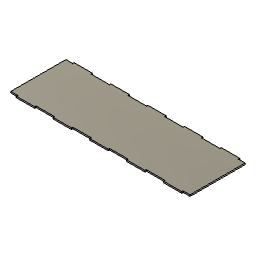
Banda version 2 v3 (Autodesk Fusion 360 archive; units mm, degrees)
design "Parte Superior"
Autodesk Fusion 360 part; units mm, degrees
sketch "Boceto1" plane through (0, 0, 0) normal (0, 0, 1) x (1, 0, 0)
  line L0 (-195, 0) -> (-195, -60)
  line L1 (-100, -60) -> (-100, -63)
  line L2 (-100, -63) -> (-60, -63)
  line L3 (-60, -63) -> (-60, -60)
  line L4 (-60, -60) -> (-20, -60)
  line L5 (-20, -60) -> (-20, -63)
  line L6 (-20, -63) -> (0, -63)
  line L7 (0, 0) -> (-195, 0) construction
  line L8 (-100, 60) -> (-100, 63)
  line L9 (-100, 63) -> (-60, 63)
  line L10 (-20, 60) -> (-20, 63)
  line L11 (-60, 60) -> (-20, 60)
  line L12 (-60, 63) -> (-60, 60)
  line L13 (-20, 63) -> (0, 63)
  line L14 (-195, 0) -> (-195, 60)
  line L15 (0, -63) -> (0, 63) construction
  line L16 (0, -63) -> (0, 63) construction
  line L17 (-100, -60) -> (-140, -60)
  line L18 (-140, -60) -> (-140, -63)
  line L19 (-140, -63) -> (-180, -63)
  line L20 (-180, -63) -> (-180, -60)
  line L21 (-180, -60) -> (-195, -60)
  line L22 (-100, 60) -> (-140, 60)
  line L23 (-140, 60) -> (-140, 63)
  line L24 (-140, 63) -> (-180, 63)
  line L25 (-180, 63) -> (-180, 60)
  line L26 (-180, 60) -> (-195, 60)
  line L27 (60, -60) -> (20, -60)
  line L28 (100, 63) -> (60, 63)
  line L29 (60, 60) -> (20, 60)
  line L30 (0, 0) -> (195, 0) construction
  line L31 (20, 60) -> (20, 63)
  line L32 (20, 63) -> (0, 63)
  line L33 (140, -63) -> (180, -63)
  line L34 (180, -63) -> (180, -60)
  line L35 (180, -60) -> (195, -60)
  line L36 (195, 0) -> (195, -60)
  line L37 (195, 0) -> (195, 60)
  line L38 (180, 60) -> (195, 60)
  line L39 (180, 63) -> (180, 60)
  line L40 (140, 63) -> (180, 63)
  line L41 (100, -60) -> (140, -60)
  line L42 (100, -63) -> (60, -63)
  line L43 (20, -63) -> (0, -63)
  line L44 (100, 60) -> (140, 60)
  line L45 (140, 60) -> (140, 63)
  line L46 (100, -60) -> (100, -63)
  line L47 (140, -60) -> (140, -63)
  line L48 (20, -63) -> (20, -60)
  line L49 (60, -63) -> (60, -60)
  line L50 (100, 63) -> (100, 60)
  line L51 (60, 63) -> (60, 60)
  point P0 (0, 63)
  dimension "d2" = 195
  dimension "d4" = 20
  dimension "d6" = 40
  dimension "d7" = 3
  dimension "d8" = 3
  dimension "d9" = 3
  dimension "d10" = 60
  dimension "d13" = 40
  dimension "d14" = 40
  dimension "d15" = 3
  dimension "d16" = 40
  dimension "d17" = 3
  dimension "d18" = 40
  dimension "d19" = 3
  dimension "d20" = 40
  dimension "d21" = 3
  constraint vertical L0
  constraint perpendicular L1 L2
  constraint perpendicular L2 L3
  constraint perpendicular L3 L4
  constraint perpendicular L4 L5
  constraint perpendicular L5 L6
  constraint coincident L7.start L30.start
  constraint perpendicular L0 L7
  constraint symmetric L0.start L7 L14.start
  constraint symmetric L0.end L7 L14.end
  constraint symmetric L1.start L7 L8.start
  constraint symmetric L1.end L7 L8.end
  constraint symmetric L2.end L7 L9.end
  constraint symmetric L3.end L7 L11.start
  constraint symmetric L4.end L7 L10.start
  constraint symmetric L5.end L7 L10.end
  constraint symmetric P0 L15 L13.end
  constraint perpendicular L1 L17
  constraint perpendicular L17 L18
  constraint perpendicular L18 L19
  constraint perpendicular L19 L20
  constraint perpendicular L0 L21
  constraint perpendicular L8 L22
  constraint perpendicular L22 L23
  constraint perpendicular L23 L24
  constraint perpendicular L24 L25
  constraint symmetric L0.start L15 L30.end
  constraint symmetric L0.end L15 L35.end
  constraint symmetric L1.start L15 L41.start
  constraint symmetric L1.end L15 L42.start
  constraint symmetric L2.end L15 L42.end
  constraint symmetric L3.end L15 L27.start
  constraint symmetric L4.end L15 L27.end
  constraint symmetric L5.end L15 L43.start
  constraint symmetric L6.end L15 L16.start
  constraint symmetric L7.start L15 L30.start
  constraint symmetric L8.start L15 L44.start
  constraint symmetric L11.start L15 L29.start
  constraint symmetric L9.end L15 L28.end
  constraint symmetric L8.end L15 L28.start
  constraint symmetric L10.start L15 L29.end
  constraint symmetric L14.end L15 L37.end
  constraint symmetric L10.end L15 L31.end
  constraint symmetric L15 P0 L13.end
  constraint symmetric L15 L17.end L41.end
  constraint symmetric L15 L18.end L33.start
  constraint symmetric L15 L19.end L33.end
  constraint symmetric L15 L20.end L34.end
  constraint symmetric L15 L22.end L44.end
  constraint symmetric L15 L23.end L40.start
  constraint symmetric L15 L24.end L39.start
  constraint symmetric L15 L25.end L38.start
  measures "d2" distance of L0.start L7.start
  measures "d4" distance of L5.end L6.end
  measures "d6" distance of L1.end L2.end
  measures "d7" distance of L1.start L1.end
  measures "d8" distance of L2.end L3.end
  measures "d9" distance of L4.end L5.end
  measures "d10" distance of L0.start L0.end
  measures "d13" distance of L3.end L4.end
  measures "d14" distance of L1.start L17.end
  measures "d15" distance of L17.end L18.end
  measures "d16" distance of L18.end L19.end
  measures "d17" distance of L19.end L20.end
  measures "d18" distance of L8.start L22.end
  measures "d19" distance of L22.end L23.end
  measures "d20" distance of L23.end L24.end
  measures "d21" distance of L24.end L25.end
extrude "Extruir2" add sketch "Boceto1" along normal blind 3

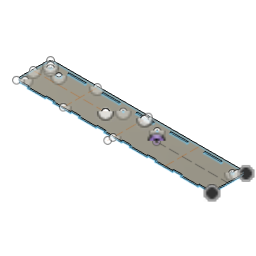
design "Lateral son motor"
Autodesk Fusion 360 part; units mm, degrees
sketch "Boceto1" plane through (0, 0, 0) normal (0, 0, 1) x (1, 0, 0)
  line L0 (-60.0005, 40.4137) -> (-60.0005, -55) construction
  line L1 (169.9995, -29.5863) -> (169.9995, 30.4137)
  line L2 (159.9995, 40.4137) -> (-60.0005, 40.4137)
  line L3 (0, 0) -> (169.9995, 0) construction
  line L4 (-0.0005, 34.4137) -> (39.9995, 34.4137)
  line L5 (39.9995, 34.4137) -> (39.9995, 31.4137)
  line L6 (39.9995, 31.4137) -> (-0.0005, 31.4137)
  line L7 (-0.0005, 31.4137) -> (-0.0005, 34.4137)
  line L8 (-60.0005, 34.4137) -> (-40.0005, 34.4137)
  line L9 (-40.0005, 34.4137) -> (-40.0005, 31.4137)
  line L10 (-40.0005, 31.4137) -> (-60.0005, 31.4137)
  circle A0 centre (-20.0005, 21.4137) radius 1
  circle A1 centre (153.9995, 24.4137) radius 2.5
  arc A2 (169.9995, 30.4137) -> (159.9995, 40.4137) centre (159.9995, 30.4137) ccw
  line L11 (79.9995, -39.5863) -> (79.9995, -42.5863)
  line L12 (79.9995, -42.5863) -> (39.9995, -42.5863)
  line L13 (39.9995, -42.5863) -> (39.9995, -39.5863)
  line L14 (39.9995, -39.5863) -> (19.9995, -39.5863)
  line L15 (19.9995, -39.5863) -> (19.9995, -42.5863)
  line L16 (19.9995, -42.5863) -> (-20.0005, -42.5863)
  line L17 (-20.0005, -42.5863) -> (-20.0005, -39.5863)
  line L18 (-20.0005, -39.5863) -> (-40.0005, -39.5863)
  line L19 (-40.0005, -39.5863) -> (-40.0005, -42.5863)
  line L20 (-40.0005, -42.5863) -> (-60.0005, -42.5863)
  line L21 (79.9995, -39.5863) -> (99.9995, -39.5863)
  line L22 (99.9995, -39.5863) -> (99.9995, -42.5863)
  line L23 (99.9995, -42.5863) -> (139.9995, -42.5863)
  line L24 (139.9995, -42.5863) -> (139.9995, -39.5863)
  line L25 (139.9995, -39.5863) -> (159.9995, -39.5863)
  arc A3 (159.9995, -39.5863) -> (169.9995, -29.5863) centre (159.9995, -29.5863) ccw
  line L26 (59.9995, 40.4137) -> (59.9995, -39.5863) construction
  line L27 (79.9995, 31.4137) -> (119.9995, 31.4137)
  line L28 (119.9995, 31.4137) -> (119.9995, 34.4137)
  line L29 (79.9995, 34.4137) -> (79.9995, 31.4137)
  line L30 (119.9995, 34.4137) -> (79.9995, 34.4137)
  line L31 (-80.0005, -39.5863) -> (-80.0005, -42.5863)
  line L32 (-120.0005, 34.4137) -> (-160.0005, 34.4137)
  line L33 (-120.0011, 0) -> (-290.0005, 0) construction
  line L34 (-60.0005, 34.4137) -> (-80.0005, 34.4137)
  line L35 (-80.0005, -42.5863) -> (-60.0005, -42.5863)
  line L36 (-290.0005, -29.5863) -> (-290.0005, 30.4137)
  line L37 (-240.0005, 34.4137) -> (-200.0005, 34.4137)
  line L38 (-200.0005, 31.4137) -> (-240.0005, 31.4137)
  line L39 (-140.0005, -42.5863) -> (-100.0005, -42.5863)
  line L40 (-160.0005, 31.4137) -> (-120.0005, 31.4137)
  line L41 (-180.0005, 40.4137) -> (-180.0005, -39.5863) construction
  line L42 (-120.0005, 31.4137) -> (-120.0005, 34.4137)
  line L43 (-80.0005, 34.4137) -> (-80.0005, 31.4137)
  line L44 (-200.0005, 34.4137) -> (-200.0005, 31.4137)
  line L45 (-160.0005, 34.4137) -> (-160.0005, 31.4137)
  arc A4 (-280.0005, 40.4137) -> (-290.0005, 30.4137) centre (-280.0005, 30.4137) ccw
  circle A5 centre (-274.0005, 24.4137) radius 2.5
  line L46 (-240.0005, 31.4137) -> (-240.0005, 34.4137)
  line L47 (-140.0005, -39.5863) -> (-140.0005, -42.5863)
  line L48 (-160.0005, -39.5863) -> (-140.0005, -39.5863)
  line L49 (-160.0005, -42.5863) -> (-160.0005, -39.5863)
  line L50 (-100.0005, -42.5863) -> (-100.0005, -39.5863)
  line L51 (-200.0005, -42.5863) -> (-160.0005, -42.5863)
  line L52 (-220.0005, -39.5863) -> (-220.0005, -42.5863)
  line L53 (-200.0005, -39.5863) -> (-220.0005, -39.5863)
  line L54 (-280.0005, 40.4137) -> (-60.0005, 40.4137)
  line L55 (-200.0005, -39.5863) -> (-200.0005, -42.5863)
  line L56 (-100.0005, -39.5863) -> (-80.0005, -39.5863)
  line L57 (-260.0005, -39.5863) -> (-280.0005, -39.5863)
  line L58 (-260.0005, -42.5863) -> (-260.0005, -39.5863)
  arc A6 (-290.0005, -29.5863) -> (-280.0005, -39.5863) centre (-280.0005, -29.5863) ccw
  line L59 (-220.0005, -42.5863) -> (-260.0005, -42.5863)
  line L60 (-80.0005, 31.4137) -> (-60.0005, 31.4137)
  circle A7 centre (-100.0005, 21.4137) radius 1
  circle A8 centre (-247.8005, 17.7137) radius 5
  point P0 (169.9995, -39.5863)
  point P1 (169.9995, 40.4137)
  point P2 (-120.0011, 0)
  point P3 (-290.0005, 40.4137)
  point P4 (-290.0005, -39.5863)
  point P5 (-120.0011, 0)
  dimension "d4" = 80
  dimension "d16" = 40
  dimension "d18" = 6
  dimension "d26" = 3
  dimension "d30" = 6
  dimension "d36" = 2
  dimension "d37" = 19
  dimension "d39" = 5
  dimension "d41" = 16
  dimension "d46" = 10
  dimension "d57" = 3
  dimension "d58" = 40
  dimension "d59" = 3
  dimension "d60" = 20
  dimension "d61" = 3
  dimension "d62" = 40
  dimension "d63" = 3
  dimension "d64" = 20
  dimension "d65" = 3
  dimension "d66" = 230
  dimension "d69" = 20
  dimension "d70" = 20
  dimension "d71" = 3
  dimension "d72" = 40
  dimension "d73" = 3
  dimension "d74" = 10
  dimension "d75" = 20
  dimension "d76" = 3
  dimension "d77" = 20
  dimension "d78" = 20
  dimension "d79" = 40
  dimension "d80" = 20
  dimension "d81" = 16
  dimension "d82" = 10
  dimension "d83" = 42.2
  dimension "d84" = 22.7
  constraint vertical L0
  constraint perpendicular L0 L2
  constraint coincident L3.start origin
  constraint horizontal L3
  constraint horizontal L4
  constraint vertical L5
  constraint horizontal L6
  constraint vertical L7
  constraint horizontal L8
  constraint vertical L9
  constraint horizontal L10
  constraint coincident L0 L8.start
  constraint symmetric L3.start L0 P5
  constraint coincident L1 L3.end
  constraint coincident P1 L2
  constraint coincident P1 L1
  constraint tangent L2 A2
  constraint tangent L1 A2
  constraint coincident P0 L1
  constraint perpendicular L11 L12
  constraint perpendicular L12 L13
  constraint perpendicular L13 L14
  constraint perpendicular L14 L15
  constraint perpendicular L15 L16
  constraint perpendicular L16 L17
  constraint perpendicular L17 L18
  constraint perpendicular L18 L19
  constraint coincident L0 L20.end
  constraint perpendicular L0 L20
  constraint perpendicular L11 L21
  constraint perpendicular L21 L22
  constraint perpendicular L22 L23
  constraint perpendicular L23 L24
  constraint perpendicular L24 L25
  constraint tangent L25 A3
  constraint tangent L1 A3
  constraint coincident L2 L26.start
  constraint coincident L21 L26.end
  constraint perpendicular L21 L26
  constraint symmetric L4.start L26 L28.end
  constraint symmetric L4.end L26 L29.start
  constraint symmetric L5.end L26 L27.start
  constraint symmetric L6.end L26 L27.end
  constraint symmetric L2.end L0 L54.end
  constraint symmetric L0 P0 P4
  constraint symmetric L0 P1 P3
  constraint symmetric L0 L3.start P2
  constraint symmetric L0 L3.end L33.end
  constraint symmetric L0 L11.start L53.start
  constraint symmetric L0 L4.start L32.start
  constraint symmetric L0 L4.end L32.end
  constraint symmetric L0 L5.end L40.start
  constraint symmetric L0 L6.end L40.end
  constraint symmetric L0 L8.start L34.start
  constraint symmetric L0 L8.end L34.end
  constraint symmetric L0 L9.end L43.end
  constraint symmetric L0 L10.end L60.end
  constraint symmetric L0 A0 A7
  constraint symmetric L0 A1 A5
  constraint symmetric L0 L2.start A4.start
  constraint symmetric L0 L1.end L36.end
  constraint symmetric L0 A2 A4
  constraint symmetric L0 L11.end L51.start
  constraint symmetric L0 L12.end L49.start
  constraint symmetric L0 L13.end L48.start
  constraint symmetric L0 L14.end L47.start
  constraint symmetric L0 L15.end L39.start
  constraint symmetric L0 L16.end L39.end
  constraint symmetric L0 L17.end L50.end
  constraint symmetric L0 L18.end L31.start
  constraint symmetric L0 L19.end L31.end
  constraint symmetric L0 L20.end L35.end
  constraint symmetric L0 L21.end L52.start
  constraint symmetric L0 L22.end L52.end
  constraint symmetric L0 L23.end L58.start
  constraint symmetric L0 L24.end L57.start
  constraint symmetric L0 L25.end L57.end
  constraint symmetric L0 L1.start L36.start
  constraint symmetric L0 A3 A6
  constraint symmetric L0 L26.start L41.start
  constraint symmetric L0 L26.end L41.end
  constraint symmetric L0 L29.start L37.end
  constraint symmetric L0 L27.end L38.end
  constraint symmetric L0 L27.start L38.start
  constraint symmetric L0 L28.end L37.start
  measures "d4" distance of P0 P1
  measures "d16" distance of L4.start L4.end
  measures "d18" distance of L2 L4
  measures "d26" distance of L4.end L5.end
  measures "d30" distance of L2 L8
  measures "d36" diameter of A0
  measures "d37" distance of L2 A0.centre
  measures "d39" diameter of A1
  measures "d41" distance of L2 A1.centre
  measures "d46" radius of A2
  measures "d57" distance of L11.start L11.end
  measures "d58" distance of L11.end L12.end
  measures "d59" distance of L12.end L13.end
  measures "d60" distance of L13.end L14.end
  measures "d61" distance of L14.end L15.end
  measures "d62" distance of L15.end L16.end
  measures "d63" distance of L16.end L17.end
  measures "d64" distance of L17.end L18.end
  measures "d65" distance of L18.end L19.end
  measures "d66" distance of L0 L1
  measures "d69" distance of L19.end L20.end
  measures "d70" distance of L11.start L21.end
  measures "d71" distance of L21.end L22.end
  measures "d72" distance of L22.end L23.end
  measures "d73" distance of L23.end L24.end
  measures "d74" radius of A3
  measures "d75" distance of L8.start L8.end
  measures "d76" distance of L8.end L9.end
  measures "d77" distance of L9.end L10.end
  measures "d78" distance of L9 A0.centre
  measures "d79" distance of L7 L9
  measures "d80" distance of L5 L26
  measures "d81" distance of L1 A1.centre
  measures "d82" diameter of A8
  measures "d83" distance of L36 A8.centre
  measures "d84" distance of L54 A8.centre
extrude "Extruir7" add sketch "Boceto1" along normal blind 3

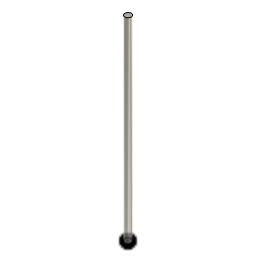
design "Barilla"
Autodesk Fusion 360 part; units mm, degrees
sketch "Boceto1" plane through (0, 0, 0) normal (0, 0, 1) x (1, 0, 0)
  circle A0 centre (0, 0) radius 2.5
  dimension "d1" = 5
  constraint coincident A0.centre origin
  measures "d1" diameter of A0
extrude "Extruir3" add sketch "Boceto1" along normal blind 150
